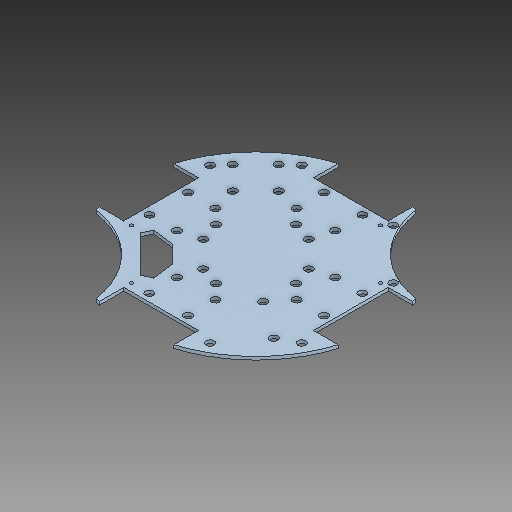
# Autodesk Inventor part: motherBoard_ыефтв
Saved by Autodesk Inventor 2020 (Build 240168000, 168)
## iProperties
Created: 2024-09-19
Part Number: motherBoard_ыефтв
Material: Типовые
Document SubType Name: Modeling
Designer: Ivan
Density: 1 g/cm^3
Appearance: Синий стальной
Author: Ivan
Autodesk Inventor part; units mm, degrees
ref_plane "YZ Plane" through (0, 0, 0) normal (1, 0, 0) x (0, 1, 0)
ref_plane "XZ Plane" through (0, 0, 0) normal (0, 1, 0) x (-1, 0, 0)
ref_plane "XY Plane" through (0, 0, 0) normal (0, 0, 1) x (1, 0, 0)
sketch "Эскиз3" plane through (0, 0, 0) normal (0, 1, 0) x (-1, 0, 0)
  line L0 (-54.5982, 80.4592) -> (-22.4528, 48.3138) construction
  line L1 (-22.4528, 48.3138) -> (-48.3138, 22.4528) construction
  line L2 (-48.3138, 22.4528) -> (-80.4592, 54.5982) construction
  line L3 (-80.4592, 54.5982) -> (-54.5982, 80.4592) construction
  line L4 (32.5269, -55.8614) -> (55.8614, -32.5269) construction
  line L5 (55.8614, -32.5269) -> (79.196, -55.8614) construction
  line L6 (79.196, -55.8614) -> (55.8614, -79.196) construction
  line L7 (55.8614, -79.196) -> (32.5269, -55.8614) construction
  circle A0 centre (0, 0) radius 20
  circle A1 centre (16, -72.43) radius 1.5
  circle A2 centre (16, -49.72) radius 1.5
  circle A3 centre (49.72, -16) radius 1.5
  circle A4 centre (49.72, 16) radius 1.5
  circle A5 centre (72.43, 31) radius 1.5
  circle A6 centre (-44.87, 82.9015) radius 1.5
  circle A7 centre (31, 72.43) radius 1.5
  circle A8 centre (72.43, 16) radius 1.5
  circle A9 centre (-49.72, 16) radius 1.5
  circle A10 centre (-49.72, -16) radius 1.5
  circle A11 centre (-16, -49.72) radius 1.5
  circle A12 centre (-16, -72.43) radius 1.5
  circle A13 centre (-72.43, -31) radius 1.5
  circle A14 centre (72.43, -16) radius 1.5
  circle A15 centre (16, 49.72) radius 1.5
  circle A16 centre (-82.9015, 44.87) radius 1.5
  circle A17 centre (-16, 72.43) radius 1.5
  circle A18 centre (44.87, -82.9015) radius 1.5
  circle A19 centre (16, 72.43) radius 1.5
  circle A20 centre (-16, 49.72) radius 1.5
  circle A21 centre (-72.43, 16) radius 1.5
  circle A22 centre (-72.43, -16) radius 1.5
  circle A23 centre (-31, -72.43) radius 1.5
  circle A24 centre (82.9015, -44.87) radius 1.5
  arc A25 (-34.57, -98.0863) -> (-98.0863, -34.57) centre (-109.0212, -109.0212) ccw
  arc A26 (-34.57, -98.0863) -> (-31, -99.2724) centre (0, 0) ccw
  line L8 (-31, -99.2724) -> (-31, -78.7724)
  line L9 (-31, -78.7724) -> (31, -78.7724)
  line L10 (31, -78.7724) -> (31, -99.2724)
  arc A27 (31, -99.2724) -> (99.2724, -31) centre (0, 0) ccw
  line L11 (99.2724, -31) -> (78.7724, -31)
  line L12 (78.7724, -31) -> (78.7724, 31)
  line L13 (78.7724, 31) -> (99.2724, 31)
  arc A28 (99.2724, 31) -> (98.0863, 34.57) centre (0, 0) ccw
  arc A29 (34.57, 98.0863) -> (98.0863, 34.57) centre (109.0212, 109.0212) ccw
  arc A30 (34.57, 98.0863) -> (31, 99.2724) centre (0, 0) ccw
  line L14 (31, 99.2724) -> (31, 78.7724)
  line L15 (31, 78.7724) -> (-31, 78.7724)
  line L16 (-31, 78.7724) -> (-31, 99.2724)
  arc A31 (-31, 99.2724) -> (-99.2724, 31) centre (0, 0) ccw
  line L17 (-99.2724, 31) -> (-78.7724, 31)
  line L18 (-78.7724, 31) -> (-78.7724, -31)
  line L19 (-78.7724, -31) -> (-99.2724, -31)
  arc A32 (-99.2724, -31) -> (-98.0863, -34.57) centre (0, 0) ccw
  line L20 (49.72, -49.72) -> (-49.72, -49.72)
  line L21 (-49.72, -49.72) -> (-49.72, 49.72)
  line L22 (-49.72, 49.72) -> (49.72, 49.72)
  line L23 (49.72, 49.72) -> (49.72, -49.72)
  line L24 (72.43, 16) -> (49.72, 16) construction
  line L25 (16, -72.43) -> (16, -49.72) construction
  line L26 (-72.43, 16) -> (-49.72, 16) construction
  line L27 (16, 72.43) -> (16, 49.72) construction
  line L28 (49.72, -49.72) -> (-49.72, 49.72) construction
  dimension "d36" = 99.44
  dimension "d37" = 32
  dimension "d38" = 32
  dimension "d39" = 32
  dimension "d40" = 32
  constraints: 58 end point, 33 centre point, 16 point on circle, 8 point on line, 5 perpendicular, 2 collinear, 2 horizontal, 2 parallel, 1 coincident, 1 midpoint, 2 other
  measures "d36" distance of L21.end L22.end
  measures "d37" distance of A3.centre L24.end
  measures "d38" distance of A11.centre L25.end
  measures "d39" distance of A10.centre L26.end
  measures "d40" distance of A20.centre L27.end
extrude "Выдавливание1" add sketch "Эскиз3" along normal blind 2.66 contours A0 | A2 L20 A11 L21 A10 A9 L22 A20 A15 L23 A4 A3 | A25 A32 L19 L18 L17 A31 L16 L15 L14 A30 A29 A28 L13 L12 L11 A27 L10 L9 L8 A26
sketch "Эскиз5" plane through (0, 2.66, 0) normal (0, 1, 0) x (1, 0, 0)
  line L0 (31, 78.7724) -> (-31, 78.7724) projected
  line L1 (-31, 78.7724) -> (-31, 99.2724) projected
  arc A0 (-31, 99.2724) -> (-99.2724, 31) centre (0, 0) ccw projected
  line L2 (-99.2724, 31) -> (-78.7724, 31) projected
  line L3 (-78.7724, 31) -> (-78.7724, -31) projected
  line L4 (-78.7724, -31) -> (-99.2724, -31) projected
  arc A1 (-99.2724, -31) -> (-98.0863, -34.57) centre (0, 0) ccw projected
  arc A2 (-34.57, -98.0863) -> (-98.0863, -34.57) centre (-109.0212, -109.0212) ccw projected
  arc A3 (-34.57, -98.0863) -> (-31, -99.2724) centre (0, 0) ccw projected
  line L5 (-31, -99.2724) -> (-31, -78.7724) projected
  line L6 (-31, -78.7724) -> (31, -78.7724) projected
  line L7 (31, -78.7724) -> (31, -99.2724) projected
  arc A4 (31, -99.2724) -> (99.2724, -31) centre (0, 0) ccw projected
  line L8 (99.2724, -31) -> (78.7724, -31) projected
  line L9 (78.7724, -31) -> (78.7724, 31) projected
  line L10 (78.7724, 31) -> (99.2724, 31) projected
  arc A5 (99.2724, 31) -> (98.0863, 34.57) centre (0, 0) ccw projected
  arc A6 (34.57, 98.0863) -> (98.0863, 34.57) centre (109.0212, 109.0212) ccw projected
  arc A7 (34.57, 98.0863) -> (31, 99.2724) centre (0, 0) ccw projected
  line L11 (31, 99.2724) -> (31, 78.7724) projected
  circle A8 centre (31, 72.43) radius 1.5 construction
  circle A9 centre (72.43, -16) radius 1.5 projected
  circle A10 centre (-16, -72.43) radius 1.5 projected
  circle A11 centre (-16, -49.72) radius 1.5 projected
  circle A12 centre (72.43, 31) radius 1.5 projected
  circle A13 centre (16, 49.72) radius 1.5 projected
  circle A14 centre (49.72, -16) radius 1.5 projected
  circle A15 centre (-16, 72.43) radius 1.5 projected
  circle A16 centre (-16, 49.72) radius 1.5 projected
  circle A17 centre (-49.72, 16) radius 1.5 projected
  circle A18 centre (-49.72, -16) radius 1.5 projected
  circle A19 centre (-72.43, -31) radius 1.5 projected
  circle A20 centre (-31, -72.43) radius 1.5 projected
  circle A21 centre (-72.43, -16) radius 1.5 projected
  circle A22 centre (49.72, 16) radius 1.5 projected
  circle A23 centre (16, 72.43) radius 1.5 projected
  circle A24 centre (-72.43, 16) radius 1.5 projected
  circle A25 centre (16, -72.43) radius 1.5 projected
  circle A26 centre (16, -49.72) radius 1.5 projected
  circle A27 centre (72.43, 16) radius 1.5 projected
  circle A28 centre (82.9015, -44.87) radius 1.5 projected
  circle A29 centre (-82.9015, 44.87) radius 1.5 projected
  circle A30 centre (-44.87, 82.9015) radius 1.5 projected
  circle A31 centre (44.87, -82.9015) radius 1.5 projected
  circle A32 centre (-31, -72.43) radius 3.3 construction
  circle A33 centre (-16, -72.43) radius 3.3
  circle A34 centre (-16, -49.72) radius 1.5 projected
  circle A35 centre (-16, -49.72) radius 3.3
  circle A36 centre (-49.72, -16) radius 1.5 projected
  circle A37 centre (-49.72, -16) radius 3.3
  circle A38 centre (-49.72, 16) radius 3.3
  circle A39 centre (-72.43, -31) radius 1.5 projected
  circle A40 centre (-72.43, -31) radius 3.3 construction
  circle A41 centre (-72.43, -16) radius 1.5 projected
  circle A42 centre (-72.43, -16) radius 3.3
  circle A43 centre (-72.43, 16) radius 1.5 projected
  circle A44 centre (-72.43, 16) radius 3.3
  circle A45 centre (-16, 49.72) radius 1.5 projected
  circle A46 centre (-16, 49.72) radius 3.3
  circle A47 centre (16, 49.72) radius 1.5 projected
  circle A48 centre (16, 49.72) radius 3.3
  circle A49 centre (49.72, 16) radius 1.5 projected
  circle A50 centre (49.72, 16) radius 3.3
  circle A51 centre (49.72, -16) radius 1.5 projected
  circle A52 centre (49.72, -16) radius 3.3
  circle A53 centre (16, -49.72) radius 1.5 projected
  circle A54 centre (16, -49.72) radius 3.3
  circle A55 centre (16, -72.43) radius 1.5 projected
  circle A56 centre (16, -72.43) radius 3.3
  circle A57 centre (44.87, -82.9015) radius 1.5 projected
  circle A58 centre (44.87, -82.9015) radius 3.3
  circle A59 centre (82.9015, -44.87) radius 1.5 projected
  circle A60 centre (82.9015, -44.87) radius 3.3
  circle A61 centre (72.43, -16) radius 3.3
  circle A62 centre (72.43, 16) radius 1.5 projected
  circle A63 centre (72.43, 16) radius 3.3
  circle A64 centre (72.43, 31) radius 1.5 projected
  circle A65 centre (72.43, 31) radius 3.3 construction
  circle A66 centre (31, 72.43) radius 3.3 construction
  circle A67 centre (16, 72.43) radius 1.5 projected
  circle A68 centre (16, 72.43) radius 3.3
  circle A69 centre (-82.9015, 44.87) radius 3.3
  circle A70 centre (-44.87, 82.9015) radius 3.3
  circle A71 centre (-16, 72.43) radius 1.5 projected
  circle A72 centre (-16, 72.43) radius 3.3
  line L12 (-55.8614, 32.5269) -> (-79.196, 55.8614) projected
  dimension "d2" = 6.6
  constraints: 24 centre point, 24 coincident, 23 equal radius
  measures "d2" diameter of A32
extrude "Выдавливание2" cut sketch "Эскиз5" against normal blind 2.66 contours A9 | A11 | A13 | A14 | A15 | A16 | A17 | A18 | A22 | A23 | A24 | A25 | A26 | A27 | A28 | A29 | A30 | A31 | A33 | A35 | A37 | A38 | A42 | A44 | A46 | A48 | A50 | A52 | A54 | A56 | A58 | A60 | A61 | A63 | A68 | A69 | A70 | A72
sketch "Эскиз6" plane through (0, 2.66, 0) normal (0, 1, 0) x (1, 0, 0)
  circle A0 centre (-72.43, -16) radius 3.3 construction
  circle A1 centre (-16, -72.43) radius 3.3 construction
  line L0 (-72.43, -31) -> (-72.43, -16) construction
  line L1 (-31, -72.43) -> (-16, -72.43) construction
  line L2 (-32.6924, -63.2376) -> (-63.2376, -32.6924)
  circle A2 centre (-16, -49.72) radius 3.3 construction
  circle A3 centre (-49.72, -16) radius 3.3 construction
  line L3 (-16, -42.22) -> (-42.22, -16) construction
  line L4 (-42.0023, -27.4404) -> (-59.5377, -25.1696)
  line L5 (-27.4404, -42.0023) -> (-25.1696, -59.5377)
  line L6 (-63.2376, -32.6924) -> (-59.5377, -25.1696) construction
  line L7 (-32.6924, -63.2376) -> (-25.1696, -59.5377) construction
  line L8 (-27.4404, -42.0023) -> (-42.0023, -27.4404) construction
  line L9 (-27.4404, -42.0023) -> (-42.0023, -27.4404)
  line L10 (-59.5377, -25.1696) -> (-63.2376, -32.6924)
  line L11 (-32.6924, -63.2376) -> (-25.1696, -59.5377)
  line L12 (32.6924, 63.2376) -> (63.2376, 32.6924)
  line L13 (42.0023, 27.4404) -> (59.5377, 25.1696)
  line L14 (63.2376, 32.6924) -> (59.5377, 25.1696)
  line L15 (32.6924, 63.2376) -> (25.1696, 59.5377)
  line L16 (27.4404, 42.0023) -> (25.1696, 59.5377)
  line L17 (27.4404, 42.0023) -> (42.0023, 27.4404)
  circle A4 centre (-72.43, -31) radius 1.5 projected
  point P0 (0, 0)
  point P1 (-23.5, -72.43)
  point P2 (-72.43, -23.5)
  point P3 (-29.11, -29.11)
  point P4 (72.43, 23.5)
  point P5 (23.5, 72.43)
  point P6 (29.11, 29.11)
  dimension "d7" = 13
  dimension "d8" = 13
  dimension "d9" = 13
  dimension "d10" = 13
  dimension "d11" = 13
  dimension "d12" = 13
  dimension "d15" = 360
  constraints: 36 end point, 12 point on line, 3 midpoint, 2 collinear, 1 horizontal, 1 vertical, 1 other
  measures "d7" distance of L2.end point (-72.43, -23.5)
  measures "d8" distance of L4.end point (-72.43, -23.5)
  measures "d9" distance of L2.start point (-23.5, -72.43)
  measures "d10" distance of L5.end point (-23.5, -72.43)
  measures "d11" distance of L5.start point (-29.11, -29.11)
  measures "d12" distance of L4.start point (-29.11, -29.11)
extrude "Выдавливание3" cut sketch "Эскиз6" against normal blind 2.66 contours L2 L10 L4 L9 L5 L11
sketch "Эскиз7" plane through (0, 2.66, 0) normal (0, 1, 0) x (1, 0, 0)
  line L0 (-42.0023, -27.4404) -> (-27.4404, -42.0023) projected
  line L1 (-27.4404, -42.0023) -> (-25.1696, -59.5377) projected
  line L2 (-25.1696, -59.5377) -> (-32.6924, -63.2376) projected
  line L3 (-32.6924, -63.2376) -> (-63.2376, -32.6924) projected
  line L4 (-63.2376, -32.6924) -> (-59.5377, -25.1696) projected
  line L5 (-59.5377, -25.1696) -> (-42.0023, -27.4404) projected
  circle A0 centre (-72.43, 16) radius 3.3 projected
  circle A1 centre (44.87, -82.9015) radius 3.3 projected
  circle A2 centre (49.72, 16) radius 3.3 projected
  circle A3 centre (-44.87, 82.9015) radius 3.3 projected
  circle A4 centre (-49.72, 16) radius 3.3 projected
  circle A5 centre (-82.9015, 44.87) radius 3.3 projected
  circle A6 centre (-16, 49.72) radius 3.3 projected
  circle A7 centre (72.43, -16) radius 3.3 projected
  circle A8 centre (16, -72.43) radius 3.3 projected
  circle A9 centre (-16, -72.43) radius 3.3 projected
  circle A10 centre (-49.72, -16) radius 3.3 projected
  circle A11 centre (16, -49.72) radius 3.3 projected
  circle A12 centre (16, 49.72) radius 3.3 projected
  circle A13 centre (16, 72.43) radius 3.3 projected
  circle A14 centre (49.72, -16) radius 3.3 projected
  circle A15 centre (72.43, 16) radius 3.3 projected
  circle A16 centre (-16, 72.43) radius 3.3 projected
  circle A17 centre (82.9015, -44.87) radius 3.3 projected
  circle A18 centre (-16, -49.72) radius 3.3 projected
  circle A19 centre (-72.43, -16) radius 3.3 projected
  line L6 (31, 78.7724) -> (-31, 78.7724) projected
  line L7 (-31, 78.7724) -> (-31, 99.2724) projected
  arc A20 (-31, 99.2724) -> (-99.2724, 31) centre (0, 0) ccw projected
  line L8 (-99.2724, 31) -> (-78.7724, 31) projected
  line L9 (-78.7724, 31) -> (-78.7724, -31) projected
  line L10 (-78.7724, -31) -> (-99.2724, -31) projected
  arc A21 (-99.2724, -31) -> (-98.0863, -34.57) centre (0, 0) ccw projected
  arc A22 (-34.57, -98.0863) -> (-98.0863, -34.57) centre (-109.0212, -109.0212) ccw projected
  arc A23 (-34.57, -98.0863) -> (-31, -99.2724) centre (0, 0) ccw projected
  line L11 (-31, -99.2724) -> (-31, -78.7724) projected
  line L12 (-31, -78.7724) -> (31, -78.7724) projected
  line L13 (31, -78.7724) -> (31, -99.2724) projected
  arc A24 (31, -99.2724) -> (99.2724, -31) centre (0, 0) ccw projected
  line L14 (99.2724, -31) -> (78.7724, -31) projected
  line L15 (78.7724, -31) -> (78.7724, 31) projected
  line L16 (78.7724, 31) -> (99.2724, 31) projected
  arc A25 (99.2724, 31) -> (98.0863, 34.57) centre (0, 0) ccw projected
  arc A26 (34.57, 98.0863) -> (98.0863, 34.57) centre (109.0212, 109.0212) ccw projected
  arc A27 (34.57, 98.0863) -> (31, 99.2724) centre (0, 0) ccw projected
  line L17 (31, 99.2724) -> (31, 78.7724) projected
  circle A28 centre (31, 72.43) radius 1.5 projected
  circle A29 centre (72.43, 31) radius 1.5 projected
  circle A30 centre (-72.43, -31) radius 1.5 projected
  circle A31 centre (-31, -72.43) radius 1.5 projected
  line L18 (31, 78.7724) -> (78.7724, 31) construction
  circle A32 centre (31, 72.43) radius 3.5 construction
  circle A33 centre (72.43, 31) radius 1.5 construction
  circle A34 centre (72.43, 31) radius 3.5 construction
  arc A35 (35.3732, 74.3992) -> (74.3992, 35.3732) centre (63.1933, 63.1933) ccw construction
  line L19 (-47.0226, -10.253) -> (10.253, 47.0226) construction
  line L20 (10.253, 47.0226) -> (47.0226, 10.253) construction
  line L21 (47.0226, 10.253) -> (-10.253, -47.0226) construction
  line L22 (-10.253, -47.0226) -> (-47.0226, -10.253) construction
  line L23 (-47.0226, -10.253) -> (47.0226, 10.253) construction
  dimension "d19" = 7
  dimension "d20" = 7
  dimension "d21" = 81
  dimension "d22" = 52
  constraints: 12 end point, 3 centre point, 3 coincident, 2 parallel, 2 point on circle, 2 point on line, 2 tangent, 1 midpoint, 1 perpendicular
  measures "d19" diameter of A32
  measures "d20" diameter of A34
  measures "d21" distance of L20.end L21.end
  measures "d22" distance of L19.end L20.end
sketch "Эскиз9" plane through (0, 2.66, 0) normal (0, 1, 0) x (1, 0, 0)
  circle A0 centre (0, 0) radius 20
  circle A1 centre (16, -72.43) radius 1.5
  circle A2 centre (16, -42.22) radius 1.5
  circle A3 centre (42.22, -16) radius 1.5
  circle A4 centre (42.22, 16) radius 1.5
  circle A5 centre (72.43, 31) radius 1.5
  circle A6 centre (-44.87, 82.9015) radius 1.5
  circle A7 centre (31, 72.43) radius 1.5
  circle A8 centre (72.43, 16) radius 1.5
  circle A9 centre (-42.22, 16) radius 1.5
  circle A10 centre (-42.22, -16) radius 1.5
  circle A11 centre (-16, -42.22) radius 1.5
  circle A12 centre (-16, -72.43) radius 1.5
  circle A13 centre (-72.43, -31) radius 1.5
  circle A14 centre (72.43, -16) radius 1.5
  circle A15 centre (16, 42.22) radius 1.5
  circle A16 centre (-82.9015, 44.87) radius 1.5
  circle A17 centre (-16, 72.43) radius 1.5
  circle A18 centre (44.87, -82.9015) radius 1.5
  circle A19 centre (16, 72.43) radius 1.5
  circle A20 centre (-16, 42.22) radius 1.5
  circle A21 centre (-72.43, 16) radius 1.5
  circle A22 centre (-72.43, -16) radius 1.5
  circle A23 centre (-31, -72.43) radius 1.5
  circle A24 centre (82.9015, -44.87) radius 1.5
  arc A25 (-34.57, -98.0863) -> (-98.0863, -34.57) centre (-109.0212, -109.0212) ccw
  arc A26 (-34.57, -98.0863) -> (-31, -99.2724) centre (0, 0) ccw
  line L0 (-31, -99.2724) -> (-31, -78.7724)
  line L1 (-31, -78.7724) -> (31, -78.7724)
  line L2 (31, -78.7724) -> (31, -99.2724)
  arc A27 (31, -99.2724) -> (99.2724, -31) centre (0, 0) ccw
  line L3 (99.2724, -31) -> (78.7724, -31)
  line L4 (78.7724, -31) -> (78.7724, 31)
  line L5 (78.7724, 31) -> (99.2724, 31)
  arc A28 (99.2724, 31) -> (98.0863, 34.57) centre (0, 0) ccw
  arc A29 (34.57, 98.0863) -> (98.0863, 34.57) centre (109.0212, 109.0212) ccw
  arc A30 (34.57, 98.0863) -> (31, 99.2724) centre (0, 0) ccw
  line L6 (31, 99.2724) -> (31, 78.7724)
  line L7 (31, 78.7724) -> (-31, 78.7724)
  line L8 (-31, 78.7724) -> (-31, 99.2724)
  arc A31 (-31, 99.2724) -> (-99.2724, 31) centre (0, 0) ccw
  line L9 (-99.2724, 31) -> (-78.7724, 31)
  line L10 (-78.7724, 31) -> (-78.7724, -31)
  line L11 (-78.7724, -31) -> (-99.2724, -31)
  arc A32 (-99.2724, -31) -> (-98.0863, -34.57) centre (0, 0) ccw
  circle A33 centre (-27.2915, 48.1257) radius 1.397 construction
  circle A34 centre (-48.1257, 27.2915) radius 1.397 construction
  circle A35 centre (-27.2915, 48.1257) radius 1.397 construction
  circle A36 centre (-48.1257, 27.2915) radius 1.397 construction
  circle A37 centre (31.2924, -37.2462) radius 1.6 construction
  circle A38 centre (53.033, -67.8823) radius 1.6 construction
  circle A39 centre (31.2924, -37.2462) radius 3.3 construction
  circle A40 centre (53.033, -67.8823) radius 3.3 construction
  circle A41 centre (-27.2915, 48.1257) radius 3.3 construction
  circle A42 centre (-48.1257, 27.2915) radius 3.3 construction
  circle A43 centre (-49.72, 16) radius 3.3 projected
  line L12 (0, 0) -> (73.5391, -73.5391) construction
  arc A44 (31, -99.2724) -> (99.2724, -31) centre (0, 0) ccw projected
  circle A45 centre (37.2462, -31.2924) radius 3.3
  circle A46 centre (67.8823, -53.033) radius 3.3
  constraints: 45 centre point, 26 end point, 18 point on circle, 9 coincident, 6 equal radius, 2 symmetric about line, 2 other
extrude "Выдавливание6" cut sketch "Эскиз9" against normal through all contours A45 | A46
sketch "Эскиз11" plane through (0, 2.66, 0) normal (0, 1, 0) x (1, 0, 0)
  arc A0 (-75.5134, 56.8864) -> (-75.5134, 52.6437) centre (-73.3921, 54.7651) ccw
  line L0 (-75.5134, 52.6437) -> (-57.1286, 34.259)
  arc A1 (-57.1286, 34.259) -> (-52.886, 34.259) centre (-55.0073, 36.3803) ccw
  line L1 (-52.886, 34.259) -> (-34.5012, 52.6437)
  arc A2 (-34.5012, 52.6437) -> (-34.5012, 56.8864) centre (-36.6225, 54.7651) ccw
  line L2 (-34.5012, 56.8864) -> (-52.886, 75.2712)
  arc A3 (-52.886, 75.2712) -> (-57.1286, 75.2712) centre (-55.0073, 73.1498) ccw
  line L3 (-57.1286, 75.2712) -> (-75.5134, 56.8864)
  circle A4 centre (-62.7855, 48.7546) radius 0.5
  circle A5 centre (-55.0073, 73.8569) radius 1.6
  circle A6 centre (-74.0992, 54.7651) radius 1.6
  circle A7 centre (-55.0073, 35.6732) radius 1.6
  circle A8 centre (-61.0177, 39.9158) radius 0.5
  circle A9 centre (-55.7144, 41.6836) radius 0.5
  circle A10 centre (-57.4822, 43.4513) radius 0.5
  circle A11 centre (-59.2499, 45.2191) radius 0.5
  circle A12 centre (-61.0177, 46.9869) radius 0.5
  circle A13 centre (-43.6936, 64.311) radius 0.5
  circle A14 centre (-41.9258, 62.5432) radius 0.5
  circle A15 centre (-62.7855, 41.6836) radius 0.5
  circle A16 centre (-59.2499, 38.148) radius 0.5
  circle A17 centre (-53.9466, 39.9158) radius 0.5
  circle A18 centre (-35.9154, 54.7651) radius 1.6
  circle A19 centre (-40.1581, 60.7755) radius 0.5
  circle A20 centre (-38.3903, 59.0077) radius 0.5
  circle A21 centre (-64.5532, 50.5224) radius 0.5
  circle A22 centre (-66.321, 45.2191) radius 0.5
  circle A23 centre (-64.5532, 43.4513) radius 0.5
  circle A24 centre (-68.0888, 46.9869) radius 0.5
  circle A25 centre (-69.8565, 48.7546) radius 0.5
  circle A26 centre (-71.6243, 50.5224) radius 0.5
  line L4 (-48.4368, -10.253) -> (9.5459, 47.7297)
  line L5 (-19.4454, 18.7383) -> (-73.5391, 73.5391) construction
  arc A27 (-31, 99.2724) -> (-99.2724, 31) centre (0, 0) ccw
  line L6 (31, 78.7724) -> (-31, 78.7724)
  line L7 (-78.7724, 31) -> (-31, 78.7724) construction
  circle A28 centre (-74.0992, 54.7651) radius 3.3
  circle A29 centre (-55.0073, 73.8569) radius 3.3
  circle A30 centre (-55.0073, 35.6732) radius 3.3
  circle A31 centre (-35.9154, 54.7651) radius 3.3
  circle A32 centre (-72.43, 16) radius 3.3 projected
  point P0 (-55.0073, 54.7651)
  point P1 (-55.0073, 54.7651)
  constraints: 32 centre point, 16 end point, 11 point on circle, 4 coincident, 4 equal radius, 2 point on line, 1 midpoint
extrude "Выдавливание7" cut sketch "Эскиз11" against normal through all contours L3 A28 L0 A0 | A0 L0 A28 L3 | A29 L2 A3 L3 | L3 A3 L2 A29 | A30 L1 A1 L0 | L0 A1 L1 A30 | A31 L1 A2 L2 | L2 A2 L1 A31 | A5 | A6 | A7 | A18
sketch "Эскиз12" plane through (0, 2.66, 0) normal (0, 1, 0) x (1, 0, 0)
  circle A0 centre (49.1515, 117.5129) radius 1.65
  circle A1 centre (49.1515, 117.5129) radius 3.35
  circle A2 centre (3.9014, 156.8484) radius 1.65
  circle A3 centre (80, 152.9999) radius 1.65
  circle A4 centre (34.7499, 192.3354) radius 1.65
  circle A5 centre (41.9507, 154.9241) radius 41.494
  line L0 (45.9767, 118.5821) -> (51.7025, 119.6842)
  arc A6 (39.3031, 113.5146) -> (45.9767, 118.5821) centre (26.7374, 136.9912) ccw
  arc A7 (51.7025, 119.6842) -> (59.7803, 117.456) centre (62.7338, 143.9197) ccw
  arc A8 (78.4993, 155.995) -> (82.5887, 163.3089) centre (57.5919, 172.4852) ccw
  circle A9 centre (80, 152.9999) radius 3.35
  arc A10 (81.5355, 142.4824) -> (78.2048, 150.1715) centre (55.7405, 135.8747) ccw
  arc A11 (5.402, 153.8533) -> (1.3126, 146.5394) centre (26.3095, 137.3631) ccw
  circle A12 centre (3.9014, 156.8484) radius 3.35
  arc A13 (2.3659, 167.3659) -> (5.6965, 159.6768) centre (28.1609, 173.9736) ccw
  arc A14 (32.1989, 190.1641) -> (24.1211, 192.3923) centre (21.1675, 165.9286) ccw
  circle A15 centre (34.7499, 192.3354) radius 3.35
  arc A16 (44.5983, 196.3336) -> (37.9247, 191.2662) centre (57.1641, 172.8571) ccw
  line L1 (39.3031, 113.5146) -> (59.7803, 117.456) construction
  line L2 (-47.0226, -10.253) -> (10.253, 47.0226) construction
  line L3 (2.3659, 167.3659) -> (59.7803, 117.456) construction
  line L4 (24.121, 192.3922) -> (81.5355, 142.4824) construction
  line L5 (1.3126, 146.5394) -> (44.5983, 196.3336) construction
  line L6 (82.5887, 163.3089) -> (39.3031, 113.5146) construction
  circle A17 centre (41.9507, 154.9241) radius 38.0979 construction
  line L7 (45.9767, 118.5821) -> (46.9111, 113.7277) construction
  line L8 (78.2048, 150.1715) -> (78.4993, 155.995) construction
  line L9 (41.9507, 154.9241) -> (80, 152.9999) construction
  line L10 (41.9507, 154.9241) -> (34.7499, 192.3354) construction
  line L11 (41.9507, 154.9241) -> (3.9014, 156.8484) construction
  line L12 (5.6965, 159.6768) -> (5.402, 153.8533) construction
  line L13 (32.1989, 190.1641) -> (37.9247, 191.2662) construction
  line L14 (41.9507, 154.9241) -> (49.1515, 117.5129) construction
  circle A18 centre (-37.8224, 4.5736) radius 3.3
  circle A19 centre (-4.5736, 37.8224) radius 3.3
  circle A20 centre (4.5736, -37.8224) radius 3.3
  circle A21 centre (37.8224, -4.5736) radius 3.3
  circle A22 centre (16, -49.72) radius 3.3 projected
  line L15 (-37.8224, 4.5736) -> (-4.5736, 37.8224) construction
  line L16 (4.5736, -37.8224) -> (37.8224, -4.5736) construction
  line L17 (-21.198, 21.198) -> (21.198, -21.198) construction
  line L18 (-4.5736, 37.8224) -> (37.8224, -4.5736) construction
  point P0 (0, 0)
  point P1 (-47.6168, 71.9305)
  point P2 (-60.3824, 55.6528)
  point P3 (-60.3824, 22.3934)
  point P4 (-47.6168, 6.1158)
  point P5 (2.7831, 6.1158)
  point P6 (15.5487, 22.3934)
  point P7 (15.2441, 55.8587)
  point P8 (2.9104, 71.5855)
  point P9 (0, 0)
  dimension "d41" = 82.9881
  dimension "d31" = 3.3
  dimension "d32" = 6.7
  dimension "d42" = 26.6279
  dimension "d43" = 20.4772
  dimension "d45" = 3.7148
  dimension "d48" = 33.1603
  dimension "d49" = 50.338
  dimension "d50" = 16.5802
  dimension "d51" = 25.169
  dimension "d53" = 10.4265
  dimension "d54" = 10.4265
  dimension "d55" = 10.4265
  dimension "d56" = 10.4265
  dimension "d57" = 10.4265
  dimension "d58" = 10.4265
  dimension "d61" = 59.957
  dimension "d62" = 47.021
  constraints: 36 end point, 28 point on circle, 21 centre point, 13 equal radius, 9 perpendicular, 6 coincident, 4 equal length, 4 parallel, 3 midpoint, 1 tangent, 12 other
  measures "d31" diameter of A0
  measures "d32" diameter of A1
  measures "d42" radius of A6
  measures "d43" horizontal distance of L1.end L1.start
  measures "d45" distance from line of L1 L0.start
  measures "d48" distance from line of L4 L3.start
  measures "d49" distance from line of L5 L6.start
  measures "d50" distance from line of L3 point (41.951, 154.924)
  measures "d51" distance from line of L5 point (41.951, 154.924)
  measures "d53" distance from line of L9 L6.start
  measures "d54" distance from line of L9 A10.start
  measures "d55" distance from line of L10 A14.end
  measures "d56" distance from line of L10 L5.end
  measures "d57" distance from line of L11 L3.start
  measures "d58" distance from line of L14 L1.end
  measures "d61" distance from line of L15 L16.end
  measures "d62" distance from line of L18 L15.start
extrude "Выдавливание8" cut sketch "Эскиз12" against normal through all
sketch "Эскиз13" plane through (0, 2.66, 0) normal (0, 1, 0) x (1, 0, 0)
  circle A0 centre (124.1994, 64.0459) radius 3
  circle A1 centre (30.7486, 82.7515) radius 1.5
  circle A2 centre (-72.43, -31) radius 1.5
  line L0 (-72.43, -31) -> (30.7486, 82.7515)
  line L1 (30.7486, 82.7515) -> (36.2927, 77.7227)
  circle A3 centre (36.2927, 77.7227) radius 2
  line L2 (-164.6688, -164.6688) -> (154.6363, 154.6363)
  circle A4 centre (77.7227, 36.2927) radius 2
  point P0 (0, 0)
  point P1 (0, 0)
  point P2 (129.0863, 44.2024)
  dimension "d63" = 6
  dimension "d64" = 7.485
  dimension "d65" = 4
  constraints: 6 end point, 5 centre point, 1 coincident, 1 perpendicular, 1 symmetric about line, 1 other
  measures "d63" diameter of A0
  measures "d64" distance from line of L0 L1.end
  measures "d65" diameter of A3
hole "Отверстие1" at (77.7227, 2.66, -36.2927) at (36.2927, 2.66, -77.7227) direction (0, -1, 0) diameter 6.5 end through all
sketch "Эскиз14" plane through (0, 2.66, 0) normal (0, 1, 0) x (1, 0, 0)
  line L0 (-38.2545, -11.9501) -> (-11.9501, -38.2545)
  line L1 (-11.9501, -38.2545) -> (38.2545, 11.9501)
  line L2 (38.2545, 11.9501) -> (11.9501, 38.2545)
  line L3 (11.9501, 38.2545) -> (-38.2545, -11.9501)
  line L4 (-38.2545, -11.9501) -> (38.2545, 11.9501) construction
  line L5 (-11.9501, -38.2545) -> (11.9501, 38.2545) construction
  line L6 (47.0226, 10.253) -> (-10.253, -47.0226) construction
  line L7 (37.5474, 11.9501) -> (11.9501, 37.5474)
  line L8 (11.9501, 37.5474) -> (-37.5474, -11.9501)
  line L9 (-37.5474, -11.9501) -> (-11.9501, -37.5474)
  line L10 (-11.9501, -37.5474) -> (37.5474, 11.9501)
  line L11 (37.5474, 11.9501) -> (-37.5474, -11.9501) construction
  line L12 (32.5976, 11.243) -> (-11.243, -32.5976)
  line L13 (0, 0) -> (31.7322, -31.7322) construction
  circle A0 centre (32.5976, 11.243) radius 1.5
  line L14 (0, 0) -> (31.7322, 31.7322) construction
  line L15 (0, 0) -> (-9.9, 29) construction
  circle A1 centre (11.243, 32.5976) radius 1.5
  circle A2 centre (-11.243, -32.5976) radius 1.5
  circle A3 centre (-32.5976, -11.243) radius 1.5
  point P0 (0, 0)
  point P1 (10.6773, -10.6773)
  point P2 (-4.9797, 4.9797)
  point P3 (0, 0)
  dimension "d73" = 37.2
  dimension "d74" = 71
  dimension "d77" = 36.2
  dimension "d78" = 70
  dimension "d79" = 4
  dimension "d80" = 3
  dimension "d81" = 3
  dimension "d82" = 3
  dimension "d83" = 4
  constraints: 30 end point, 7 parallel, 6 midpoint, 4 centre point, 4 coincident, 3 perpendicular, 3 symmetric about line, 2 point on line, 4 other
  measures "d73" distance of L0.start L0.end
  measures "d74" distance from line of L0 L1.end
  measures "d77" distance of L9.end L8.end
  measures "d78" distance of L8.end L7.end
  measures "d79" distance from line of L7 L12.start
  measures "d80" distance from line of L10 point (10.677, -10.677)
  measures "d81" diameter of A0
  measures "d82" distance from line of L8 A1.centre
  measures "d83" distance from line of L9 L12.end
hole "Отверстие2" at (32.5976, 2.66, -11.243) at (-11.243, 2.66, 32.5976) at (-32.5976, 2.66, 11.243) at (11.243, 2.66, -32.5976) direction (0, -1, 0) diameter 6.5 end through all
equation "\"d38\" = d37"
equation "\"d39\" = d37"
equation "\"d40\" = d37"
equation "\"d8\" = d7"
equation "\"d9\" = d7"
equation "\"d10\" = d9"
equation "\"d11\" = d7"
equation "\"d12\" = d11"
